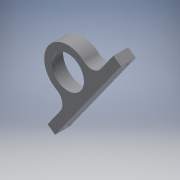
# Autodesk Inventor part: bearing block
Saved by Autodesk Inventor 2017 (Build 210142000, 142)
## iProperties
Created: 2018-11-26
Part Number: bearing block
Material: Generic
Document SubType Name: Modeling
Designer: Eric the Great
Density: 1 g/cm^3
Appearance: Default
Author: Eric the Great
Autodesk Inventor part; units mm, degrees
ref_plane "YZ Plane" through (0, 0, 0) normal (1, 0, 0) x (0, 1, 0)
ref_plane "XZ Plane" through (0, 0, 0) normal (0, 1, 0) x (-1, 0, 0)
ref_plane "XY Plane" through (0, 0, 0) normal (0, 0, 1) x (1, 0, 0)
sketch "Sketch1" plane through (0, 0, 0) normal (0, 0, 1) x (1, 0, 0)
  circle A0 centre (0, 0) radius 11 projected
  arc A1 (9.103, 9.9692) -> (-6.4691, -11.8491) centre (0, 0) ccw
  line L0 (122.2578, 146.7857) -> (-99.0763, -163.3307) projected
  arc A2 (9.103, 9.9692) -> (18.8408, 11) centre (13.515, 14.8011) ccw
  line L1 (18.8408, 11) -> (26.1613, 21.2569)
  line L2 (26.1613, 21.2569) -> (30.471, 18.181)
  line L3 (0, 0) -> (9.5455, -6.8127)
  line L4 (-7.2894, -34.726) -> (30.471, 18.181)
  arc A3 (-4.2786, -21.3932) -> (-6.4691, -11.8491) centre (-9.6045, -17.5921) ccw
  line L5 (-4.2786, -21.3932) -> (-11.5991, -31.6501)
  line L6 (-11.5991, -31.6501) -> (-7.2894, -34.726)
  line L7 (-7.2894, -34.726) -> (30.471, 18.181)
  circle A4 centre (0, 0) radius 11.25
  point P0 (0, 0)
  point P1 (-99.0763, -163.3307)
  point P2 (122.2578, 146.7857)
  dimension "d0" = 2.5
  dimension "d12" = 65
  dimension "d15" = 22.5
  constraints: 14 end point, 7 symmetric about line, 6 point on circle, 4 centre point, 2 coincident, 2 tangent, 1 parallel, 1 perpendicular, 1 point on line, 1 other
  measures "d0" radial gap between concentric circles of A1 A0
  measures "d12" distance between parallel lines of L6 L2
  measures "d15" diameter of A4
extrude "Extrusion1" add sketch "Sketch1" along normal blind 8.5 contours A2 L1 L2 L0 L6 L5 A3 A1
sketch "Sketch2" plane through (0, 0, 8.5) normal (0, 0, 1) x (1, 0, 0)
  circle A0 centre (0, 0) radius 9.2831
  circle A1 centre (0, 0) radius 10.96 projected
  circle A2 centre (0, 0) radius 13.5
  dimension "d3" = 18.5661
  constraints: 2 centre point, 2 coincident
  measures "d3" diameter of A0
extrude "Extrusion2" add sketch "Sketch2" against normal blind 1.5 contours A1 | A2
sketch "Sketch3" plane through (-11.5991, -31.6501, 0) normal (-0.8139539, 0.5809295, 0) x (0, 0, 1)
  line L0 (0, 12.6013) -> (0, 0) projected
  line L1 (0, 0) -> (8.5, 0) projected
  line L2 (8.5, 12.6013) -> (8.5, 0) projected
  line L3 (0, 12.6013) -> (8.5, 12.6013) projected
  line L4 (0, 65) -> (0, 52.3987) projected
  line L5 (0, 52.3987) -> (8.5, 52.3987) projected
  line L6 (8.5, 65) -> (8.5, 52.3987) projected
  line L7 (0, 65) -> (8.5, 65) projected
  line L8 (3.4344, 32.2582) -> (4.7482, 32.2582)
  circle A0 centre (4.25, 4) radius 1.75
  circle A1 centre (4.25, 61) radius 1.75
  point P0 (0, 32.5)
  dimension "d10" = 3.5
  dimension "d11" = 3.5
  dimension "d13" = 4
  dimension "d14" = 4
  constraints: 2 centre point, 2 end point, 1 horizontal, 1 vertical alignment
  measures "d10" diameter of A0
  measures "d11" diameter of A1
  measures "d13" distance from line of A1.centre L7
  measures "d14" distance from line of L1 A0.centre
extrude "Extrusion3" cut sketch "Sketch3" against normal up to surface (5.2948 mm away) contours A0 | A1
body "Solid1"
